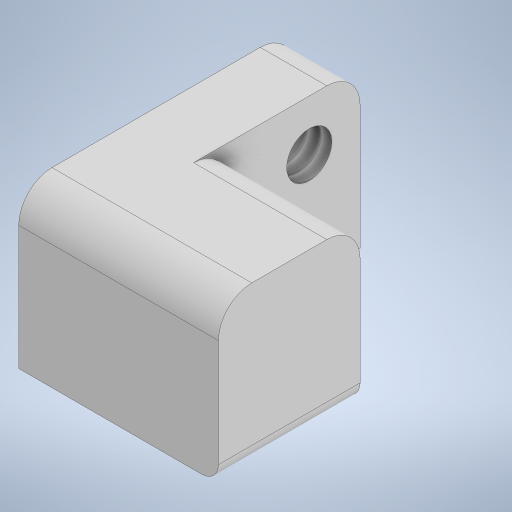
# Autodesk Inventor part: AFL-101-002-01-4E RetainerNut
Saved by Autodesk Inventor 2024.1 (Build 281209000, 209)
## iProperties
Created: 2024-12-30
Part Number: AFL-101-002-01-4E RetainerNut
Material: Generic
Document SubType Name: Modeling
Designer: pab2
Density: 1 g/cm^3
Appearance: Default
Author: pab2
Autodesk Inventor part; units mm, degrees
ref_plane "YZ Plane" through (0, 0, 0) normal (1, 0, 0) x (0, 1, 0)
ref_plane "XZ Plane" through (0, 0, 0) normal (0, 1, 0) x (-1, 0, 0)
ref_plane "XY Plane" through (0, 0, 0) normal (0, 0, 1) x (1, 0, 0)
sketch "Sketch1" plane through (0, 0, 0) normal (0, 1, 0) x (-1, 0, 0)
  line L0 (0, 0) -> (3.175, 0)
  line L1 (3.175, 0) -> (3.175, -6.35)
  line L2 (3.175, -6.35) -> (0, -6.35)
  line L3 (0, -6.35) -> (0, 0)
  line L4 (0, 0) -> (9.525, 0)
  line L5 (9.525, 0) -> (9.525, 8.255)
  line L6 (9.525, 8.255) -> (0, 8.255)
  line L7 (0, 8.255) -> (0, 0)
  line L8 (3.175, 0) -> (-6.35, 0)
  line L9 (-6.35, 0) -> (-6.35, 8.255)
  line L10 (-6.35, 8.255) -> (3.175, 8.255)
  line L11 (3.175, 8.255) -> (3.175, 0)
  dimension "d0" = 3.175
  dimension "d1" = 6.35
  dimension "d2" = 9.525
  dimension "d3" = 8.255
  dimension "d21" = 9.525
  constraints: 24 end point, 6 parallel, 3 horizontal, 3 perpendicular
  measures "d0" distance of L1.end L2.end
  measures "d1" distance of L0.end L1.end
  measures "d2" distance of L6.end L5.end
  measures "d3" distance of L5.end L4.end
  measures "d21" distance of L9.end L10.end
extrude "Extrusion1" add sketch "Sketch1" along normal blind 8.255 contours L7 L6 L11 L0 | L0 L1 L2 L3 | L8 L9 L10 L7
sketch "Sketch2" plane through (0, 0, 8.255) normal (1, 0, 0) x (0, 0, -1)
  line L0 (8.255, 8.255) -> (14.605, 8.255) projected
  line L1 (14.605, 8.255) -> (11.43, 8.255)
  line L2 (11.43, 8.255) -> (11.43, 5.08)
  line L3 (11.43, 5.08) -> (14.605, 5.08)
  line L4 (14.605, 5.08) -> (14.605, 8.255)
  point P0 (8.255, 0)
  point P1 (0, 8.255)
  dimension "d6" = 3.175
  dimension "d7" = 3.175
  constraints: 8 end point, 2 parallel, 1 horizontal, 1 perpendicular
  measures "d6" distance of L3.end L2.end
  measures "d7" distance of L2.end L1.end
hole "Hole1" at (0, 5.08, -3.175) direction (-1, 0, 0) diameter 2.1565 depth 8.8646 tip angle 118 thread size "4-40 UNC" class "2B" standard "ANSI Unified Screw Threads"
sketch "Sketch3" plane through (0, 8.255, 0) normal (0, 1, 0) x (1, 0, 0)
  line L0 (0, 0) -> (0, 6.35) projected
  line L1 (0, 6.35) -> (-3.175, 6.35) projected
  line L2 (-3.175, 6.35) -> (-3.175, -8.255) projected
  line L3 (-3.175, -8.255) -> (6.35, -8.255) projected
  line L4 (6.35, -8.255) -> (6.35, 0) projected
  line L5 (6.35, 0) -> (0, 0) projected
extrude "Extrusion2" cut sketch "Sketch3" against normal blind 0.75
sketch "Sketch4" plane through (0, 0, -6.35) normal (0, 0, -1) x (-1, 0, 0)
  line L0 (3.175, 7.505) -> (0, 7.505) projected
  line L1 (0, 0) -> (0, 7.505) projected
  line L2 (0, 0) -> (3.175, 0) projected
  line L3 (3.175, 0) -> (3.175, 7.505) projected
extrude "Extrusion3" cut sketch "Sketch4" against normal blind 0.75
sketch "Sketch5" plane through (-9.525, 0, 8.255) normal (0, 0, 1) x (1, 0, 0)
  line L0 (15.875, 7.505) -> (6.35, 7.505) projected
  line L1 (6.35, 0) -> (15.875, 0) projected
  line L2 (6.35, 0) -> (6.35, 7.505) projected
  line L3 (15.875, 0) -> (15.875, 7.505) projected
  line L4 (15.875, 7.505) -> (6.35, 7.505) projected
  line L5 (6.35, 0) -> (6.35, 7.505) projected
  line L6 (6.35, 0) -> (15.875, 0) projected
  line L7 (15.875, 0) -> (15.875, 7.505) projected
  point P0 (9.525, 0)
extrude "Extrusion4" cut sketch "Sketch5" against normal blind 0.75
sketch "Sketch6" plane through (6.35, 0, 0) normal (0, 0, -1) x (-1, 0, 0)
  line L0 (6.35, 7.505) -> (0, 7.505) projected
  line L1 (0, 0) -> (0, 7.505) projected
  line L2 (0, 0) -> (6.35, 0) projected
  line L3 (6.35, 0) -> (6.35, 7.505) projected
extrude "Extrusion5" cut sketch "Sketch6" against normal blind 0.75
fillet "Fillet1" radius 1.5875 3 edges at (1.5875, 7.505, 7.505) (-1.5875, 7.505, -5.6) (3.175, 7.505, 0.75)
fillet "Fillet2" radius 0.7937 1 edges at (6.35, 0, 4.1275)
body "Solid1"
